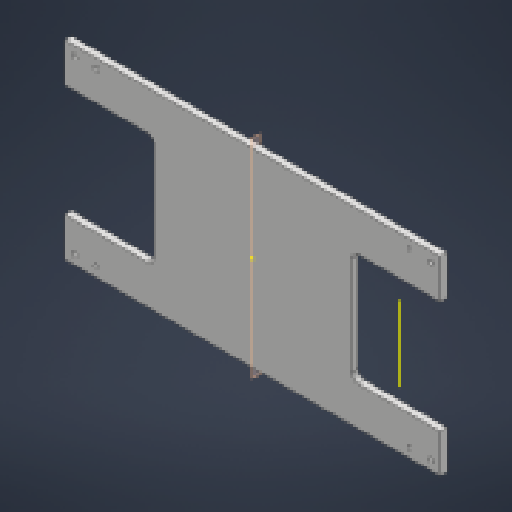
# Autodesk Inventor part: 玻纤
Saved by Autodesk Inventor 2025 (Build 290162000, 162)
## iProperties
Created: 2025-11-09
Part Number: 玻纤
Material: 常规
Document SubType Name: Modeling
Designer: XH
Density: 1 g/cm^3
Appearance: 默认
Author: XH
Autodesk Inventor part; units mm, degrees
ref_plane "YZ Plane" through (0, 0, 0) normal (1, 0, 0) x (0, 1, 0)
ref_plane "XZ Plane" through (0, 0, 0) normal (0, 1, 0) x (-1, 0, 0)
ref_plane "XY Plane" through (0, 0, 0) normal (0, 0, 1) x (1, 0, 0)
sketch "草图1" plane through (0, 0, 0) normal (0, 0, 1) x (1, 0, 0)
  line L0 (140, -71) -> (-140, -71)
  line L1 (-140, -71) -> (-140, 71)
  line L2 (-140, 71) -> (140, 71)
  line L3 (140, 71) -> (140, -71)
  line L4 (140, -71) -> (-140, 71) construction
  line L5 (-140, -71) -> (140, 71) construction
  point P0 (0, 0)
  dimension "d0" = 280
  dimension "d1" = 142
  constraints: 12 end point, 2 midpoint, 2 parallel, 1 horizontal, 1 perpendicular
  measures "d0" distance of L1.end L2.end
  measures "d1" distance of L0.end L1.end
extrude "拉伸1" add sketch "草图1" along normal blind 5
sketch "草图2" plane through (0, 0, 5) normal (0, 0, 1) x (1, 0, 0)
  line L0 (110, 27.873) -> (110, -28.2358) projected
  point P0 (0, 0)
sketch "草图3" plane through (0, 0, 5) normal (0, 0, 1) x (1, 0, 0)
  point P0 (0, 0)
sketch "草图4" plane through (0, 0, 5) normal (0, 0, 1) x (1, 0, 0)
  circle A0 centre (117, 63.8186) radius 1.85 projected
  circle A1 centre (133, 63.8186) radius 1.85 projected
  circle A2 centre (117, -64.1814) radius 1.85 projected
  circle A3 centre (133, -64.1814) radius 1.85 projected
  line L0 (140, -32.9821) -> (110, -32.9821) projected
  line L1 (110, 32.6193) -> (140, 32.6193) projected
  line L2 (140, -71) -> (140, 71) projected
  line L3 (140, -41.9821) -> (73.7163, -41.9821)
  line L4 (73.7163, -41.9821) -> (73.7163, 41.6193)
  line L5 (73.7163, 41.6193) -> (140, 41.6193)
  line L6 (140, 41.6193) -> (140, -41.9821)
  point P0 (0, 0)
  dimension "d4" = 9
  dimension "d5" = 9
  constraints: 8 end point, 2 parallel, 1 horizontal, 1 perpendicular, 1 point on line
  measures "d4" distance between parallel lines of L5 L1
  measures "d5" distance between parallel lines of L3 L0
extrude "拉伸2" cut sketch "草图4" against normal blind 5
ref_plane "工作平面1" through (0, 71, 5) normal (1, 0, 0) x (0, 0, -1)
mirror "镜像1" about plane through (0, 71, 5) normal (1, 0, 0) of "拉伸2"
fillet "圆角1" radius 5 4 edges at (73.7163, -41.9821, 2.5) (73.7163, 41.6193, 2.5) (-73.7163, 41.6193, 2.5) (-73.7163, -41.9821, 2.5)
